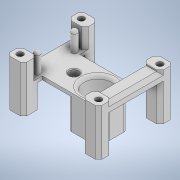
# Autodesk Inventor part: motor holder under
Saved by Autodesk Inventor 2022 (Build 260153000, 153)
## iProperties
Created: 2021-11-29
Part Number: motor holder under
Material: Generic
Document SubType Name: Modeling
Designer: Alec Warren
Density: 1 g/cm^3
Appearance: Default
Author: Alec Warren
Autodesk Inventor part; units mm, degrees
ref_plane "YZ Plane" through (0, 0, 0) normal (1, 0, 0) x (0, 1, 0)
ref_plane "XZ Plane" through (0, 0, 0) normal (0, 1, 0) x (-1, 0, 0)
ref_plane "XY Plane" through (0, 0, 0) normal (0, 0, 1) x (1, 0, 0)
sketch "Sketch1" plane through (0, 0, 0) normal (0, 1, 0) x (-1, 0, 0)
  line L0 (0, 0) -> (0, 22.5)
  line L1 (0, 22.5) -> (-41.8, 22.5)
  line L2 (-41.8, 22.5) -> (-41.8, 0)
  line L3 (-41.8, 0) -> (0, 0)
  line L4 (0, 11.25) -> (-37, 11.25)
  line L5 (-37, 11.25) -> (-41.8, 11.25)
  line L6 (-39.4, 11.25) -> (-25.4, 11.25)
  line L7 (-25.4, 11.25) -> (-14.15, 11.25)
  line L8 (-14.15, 11.25) -> (-5.55, 11.25)
  line L9 (-5.55, 11.25) -> (-5.55, 2.45)
  line L10 (-5.55, 11.25) -> (-5.55, 20.05)
  circle A0 centre (-5.55, 2.45) radius 1.375
  circle A1 centre (-5.55, 20.05) radius 1.375
  line L11 (-37, 0) -> (-37, 22.5)
  line L12 (0, 22.5) -> (0, 28.9)
  line L13 (0, 0) -> (0, -6.4)
  line L14 (0, -6.4) -> (-41.8, -6.4)
  line L15 (-41.8, -6.4) -> (-41.8, 0)
  line L16 (-41.8, 22.5) -> (-41.8, 28.9)
  line L17 (-41.8, 28.9) -> (0, 28.9)
  line L18 (0, -3.2) -> (-3.2, -3.2)
  line L19 (0, 25.7) -> (-3.2, 25.7)
  circle A2 centre (-3.2, -3.2) radius 1.6
  circle A3 centre (-25.4, 11.25) radius 6.5
  line L20 (-38.6, -3.2) -> (-3.2, -3.2)
  line L21 (-3.2, -3.2) -> (-20.9, -3.2)
  circle A4 centre (-12.05, -3.2) radius 1.6
  line L22 (-38.6, -3.2) -> (-20.9, -3.2)
  circle A5 centre (-20.9, -3.2) radius 1.6
  circle A6 centre (-29.75, -3.2) radius 1.6
  circle A7 centre (-3.2, 25.7) radius 1.6
  circle A8 centre (-14.15, 11.25) radius 2.25
  circle A9 centre (-3.2, 25.7) radius 1.45
  line L23 (-41.8, 25.7) -> (-41.8, -3.2)
  circle A10 centre (-12.05, 25.7) radius 1.45
  circle A11 centre (-20.9, 25.7) radius 1.45
  circle A12 centre (-29.75, 25.7) radius 1.45
  circle A13 centre (-38.6, 25.7) radius 1.45
  circle A14 centre (-3.2, -3.2) radius 1.45
  circle A15 centre (-12.05, -3.2) radius 1.45
  circle A16 centre (-20.9, -3.2) radius 1.45
  circle A17 centre (-29.75, -3.2) radius 1.45
  circle A18 centre (-38.6, -3.2) radius 1.45
  line L24 (-41.8, 28.9) -> (-43.4, 28.9)
  line L25 (-43.4, 28.9) -> (-43.4, -6.4)
  line L26 (-43.4, -6.4) -> (-41.8, -6.4)
  line L27 (-41.8, 22.5) -> (-43.4, 22.5)
  line L28 (-41.8, 0) -> (-43.4, 0)
  line L29 (-43.4, -3.2) -> (-40.2, -3.2)
  circle A19 centre (-40.2, -3.2) radius 1.6
  line L30 (-43.4, 25.7) -> (-40.2, 25.7)
  circle A20 centre (-40.2, 25.7) radius 1.6
  line L31 (-4.8, 25.7) -> (-8, 25.7)
  line L32 (-38.6, 25.7) -> (-35.4, 25.7)
  line L33 (-35.4, 25.7) -> (-35.4, 28.9)
  line L34 (-35.4, 22.5) -> (-35.4, 25.7)
  line L35 (-8, 25.7) -> (-8, 28.9)
  line L36 (-8, 25.7) -> (-8, 22.5)
  line L37 (-4.8, -3.2) -> (-8, -3.2)
  line L38 (-8, -3.2) -> (-8, -6.4)
  line L39 (-8, 0) -> (-8, -3.2)
  line L40 (-38.6, -3.2) -> (-35.4, -3.2)
  line L41 (-35.4, -3.2) -> (-35.4, 0)
  line L42 (-35.4, -6.4) -> (-35.4, -3.2)
  line L43 (-8, 22.5) -> (-8, 20.05)
  line L44 (-8, 0) -> (-8, 2.45)
  line L45 (-35.4, 0) -> (-35.4, 2.45)
  line L46 (-35.4, 2.45) -> (-8, 2.45)
  line L47 (-35.4, 22.5) -> (-35.4, 20.05)
  line L48 (-35.4, 20.05) -> (-8, 20.05)
  line L49 (-8, 2.45) -> (-8, 20.05)
  line L50 (-16.4, 11.25) -> (-18.9, 11.25)
  line L51 (-17.65, 11.25) -> (-17.65, 20.05)
  line L52 (-17.65, 11.25) -> (-17.65, 2.45)
  line L53 (-31.9, 11.25) -> (-34.3, 11.25)
  line L54 (-34.3, 11.25) -> (-34.3, 2.45)
  line L55 (-34.3, 11.25) -> (-34.3, 20.05)
  line L56 (-18.9, 11.25) -> (-16.5, 11.25)
  line L57 (-16.5, 11.25) -> (-16.5, 2.45)
  line L58 (-16.5, 20.05) -> (-16.5, 11.25)
  circle A21 centre (-40.2, 25.7) radius 1.45
  circle A22 centre (-40.2, -3.2) radius 1.45
  dimension "d19" = 3.2
  dimension "d35" = 4.5
  dimension "d0" = 22.5
  dimension "d1" = 41.8
  dimension "d2" = 37
  dimension "d3" = 4.8
  dimension "d4" = 14
  dimension "d5" = 11.25
  dimension "d6" = 8.6
  dimension "d7" = 8.8
  dimension "d8" = 8.8
  dimension "d9" = 2.75
  dimension "d10" = 2.75
  dimension "d12" = 6.4
  dimension "d13" = 6.4
  dimension "d15" = 3.2
  dimension "d18" = 3.2
  dimension "d23" = 13
  dimension "d24" = 3.2
  dimension "d25" = 3.2
  dimension "d26" = 3.2
  dimension "d36" = 2.9
  dimension "d37" = 28.9
  dimension "d40" = 8.85
  dimension "d43" = 28.9
  dimension "d53" = 1.6
  dimension "d58" = 3.2
  dimension "d59" = 3.2
  dimension "d60" = 3.2
  dimension "d66" = 3.2
  dimension "d67" = 3.2
  dimension "d68" = 3.2
  dimension "d69" = 3.2
  dimension "d74" = 2.4
  dimension "d86" = 2.4
  dimension "d94" = 2.9
  dimension "d95" = 2.9
  constraints: 118 end point, 39 point on line, 23 perpendicular, 20 centre point, 11 coincident, 11 midpoint, 9 horizontal, 9 vertical, 4 equal length, 3 horizontal alignment, 2 point on circle, 1 symmetric about line, 24 other
  measures "d0" distance of L0.start L0.end
  measures "d1" distance of L0.end L1.end
  measures "d2" distance of L4.start L4.end
  measures "d3" distance of L4.end L5.end
  measures "d4" distance of L6.start L6.end
  measures "d5" distance of L6.end L7.end
  measures "d6" distance of L7.end L8.end
  measures "d7" distance of L8.end L9.end
  measures "d8" distance of L8.end L10.end
  measures "d9" diameter of A0
  measures "d10" diameter of A1
  measures "d12" distance of L0.end L12.end
  measures "d13" distance of L0.start L13.end
  measures "d15" distance of L18.start L18.end
  measures "d18" distance of L19.start L19.end
  measures "d23" diameter of A3
  measures "d24" diameter of A4
  measures "d25" diameter of A5
  measures "d26" diameter of A6
  measures "d36" diameter of A9
  measures "d37" distance of L23.start L23.end
  measures "d40" distance of A9.centre A10.centre
  measures "d43" distance of A9.centre A14.centre
  measures "d53" distance of L16.end L24.end
  measures "d58" distance of L29.start L29.end
  measures "d59" distance of L30.start L30.end
  measures "d60" diameter of A20
  measures "d66" distance of L31.start L31.end
  measures "d67" distance of L32.start L32.end
  measures "d68" distance of L37.start L37.end
  measures "d69" distance of L40.start L40.end
  measures "d74" distance of L53.start L53.end
  measures "d86" distance of L50.end L56.end
  measures "d94" diameter of A21
  measures "d95" diameter of A22
extrude "Extrusion1" add sketch "Sketch1" along normal blind 3.2 contours L3 L44 L49 L4 L0 | L13 L18 A2 L20 L39 L3 | L4 L49 L43 L1 L0 | L39 L20 A4 A5 A6 L41 L3 | L13 L14 L38 L20 A2 L18 | L1 L36 L31 A7 L19 L12 | L41 L20 A18 A19 L15 L3 | L3 L11 L4 L54 L46 L45 | L38 L14 L42 L20 A6 A5 A4 | L46 L57 L4 A8 L49 | A2 L20 A14 L18 | L18 A14 L20 A2 | L1 L34 L33 L17 L35 L36 | L19 A7 L31 L35 L17 L12 | L4 A8 L58 L48 L49 | L3 L2 L5 L11 | L42 L14 L15 A19 A18 L20 | A4 L20 A15 | L20 A15 A4 | L46 L52 L4 L57 | A14 L20 L18 | L18 L20 A14 | L47 L48 L55 L4 L11 L1 | L1 L16 A20 A13 L32 L34 | A7 | L28 L25 L27 L2 | L15 L29 L25 L28 | L5 L2 L1 L11 | A18 A19 L20 | L20 A19 A18 | A6 L20 A17 | L20 A17 A6 | L54 L4 A3 L52 L46 | A15 L20 | L20 A15 | L4 L51 L48 L58 | L32 A13 A20 L16 L17 L33 | L15 L26 L25 L29 | A19 A18 A22 L29 | L29 A22 A18 A19 | L55 L48 L51 L4 A3 | A19 A18 A22 | A17 L20 | L20 A17 | A5 L20 A16 | L20 A16 A5 | L27 L25 L30 L16 | L32 A20 A13 | A13 A20 L32 | A22 A18 | A22 A18 | A16 L20 | L20 A16 | L30 L25 L24 L16 | A20 A13 A21 L30 | L30 A21 A13 A20 | A20 A13 A21 | A21 A13 | A21 A13 | A0 | A1 | A9 | A10 | A11 | A12
extrude "Extrusion2" add sketch "Sketch1" along normal blind 9.3 from surface at 3.2 contours L13 L18 A2 L20 L39 L3 | L39 L20 A4 A5 A6 L41 L3 | L13 L14 L38 L20 A2 L18 | L1 L36 L31 A7 L19 L12 | L41 L20 A18 A19 L15 L3 | L38 L14 L42 L20 A6 A5 A4 | A2 L20 A14 L18 | L18 A14 L20 A2 | L1 L34 L33 L17 L35 L36 | L19 A7 L31 L35 L17 L12 | L42 L14 L15 A19 A18 L20 | A4 L20 A15 | L20 A15 A4 | A14 L20 L18 | L18 L20 A14 | L1 L16 A20 A13 L32 L34 | A7 | A18 A19 L20 | L20 A19 A18 | A6 L20 A17 | L20 A17 A6 | A15 L20 | L20 A15 | L32 A13 A20 L16 L17 L33 | A19 A18 A22 L29 | L29 A22 A18 A19 | A19 A18 A22 | A17 L20 | L20 A17 | A5 L20 A16 | L20 A16 A5 | L32 A20 A13 | A13 A20 L32 | A22 A18 | A22 A18 | A16 L20 | L20 A16 | A20 A13 A21 L30 | L30 A21 A13 A20 | A20 A13 A21 | A21 A13 | A21 A13 | A0 | A1 | A9 | A10 | A11 | A12
extrude "Extrusion4" add sketch "Sketch1" along normal blind 8.7 from surface at 3.2 contours L3 L2 L5 L11 | L5 L2 L1 L11
fillet "Fillet2" radius 1.35 2 edges at (6.925, 12.5, 2.45) (6.925, 12.5, 20.05)
extrude "Extrusion6" add sketch "Sketch1" against normal blind 9.5 contours L13 L18 A2 L20 L39 L3 | L39 L20 A4 A5 A6 L41 L3 | L13 L14 L38 L20 A2 L18 | L1 L36 L31 A7 L19 L12 | L41 L20 A18 A19 L15 L3 | L3 L11 L4 L54 L46 L45 | L38 L14 L42 L20 A6 A5 A4 | L46 L57 L4 A8 L49 | A2 L20 A14 L18 | L18 A14 L20 A2 | L1 L34 L33 L17 L35 L36 | L19 A7 L31 L35 L17 L12 | L4 A8 L58 L48 L49 | L3 L2 L5 L11 | L42 L14 L15 A19 A18 L20 | A4 L20 A15 | L20 A15 A4 | L46 L52 L4 L57 | A14 L20 L18 | L18 L20 A14 | L47 L48 L55 L4 L11 L1 | L1 L16 A20 A13 L32 L34 | A7 | A8 L4 | L4 A8 | L28 L25 L27 L2 | L15 L29 L25 L28 | L5 L2 L1 L11 | A18 A19 L20 | L20 A19 A18 | A6 L20 A17 | L20 A17 A6 | L54 L4 A3 L52 L46 | A15 L20 | L20 A15 | L4 L51 L48 L58 | L32 A13 A20 L16 L17 L33 | L15 L26 L25 L29 | A19 A18 A22 L29 | L29 A22 A18 A19 | L55 L48 L51 L4 A3 | A19 A18 A22 | A17 L20 | L20 A17 | A5 L20 A16 | L20 A16 A5 | L27 L25 L30 L16 | L32 A20 A13 | A13 A20 L32 | A22 A18 | A22 A18 | A16 L20 | L20 A16 | L30 L25 L24 L16 | A20 A13 A21 L30 | L30 A21 A13 A20 | A20 A13 A21 | A21 A13 | A21 A13 | A9 | A10 | A11 | A12
extrude "Extrusion7" add sketch "Sketch1" along normal up to surface (12.5 mm away) contours L15 L29 L25 L28 | L15 L26 L25 L29 | L27 L25 L30 L16 | L30 L25 L24 L16
extrude "Extrusion8" add sketch "Sketch1" along normal up to surface (11.9 mm away) contours L28 L25 L27 L2
extrude "Extrusion9" cut sketch "Sketch1" against normal blind 10 from surface at 12.5 contours A14 L20 L18 | L18 L20 A14 | A22 A18 | A22 A18 | A21 A13 | A21 A13 | A9
extrude "deleting underneath" cut sketch "Sketch1" against normal through all contours L39 L20 A4 A5 A6 L41 L3 | L3 L11 L4 L54 L46 L45 | L38 L14 L42 L20 A6 A5 A4 | L46 L57 L4 A8 L49 | L1 L34 L33 L17 L35 L36 | L4 A8 L58 L48 L49 | L3 L2 L5 L11 | A4 L20 A15 | L20 A15 A4 | L47 L48 L55 L4 L11 L1 | A8 L4 | L4 A8 | L28 L25 L27 L2 | L5 L2 L1 L11 | A6 L20 A17 | L20 A17 A6 | A15 L20 | L20 A15 | A17 L20 | L20 A17 | A5 L20 A16 | L20 A16 A5 | A16 L20 | L20 A16 | A10 | A11 | A12
extrude "deleting above" cut sketch "Sketch1" along normal through all contours L39 L20 A4 A5 A6 L41 L3 | L38 L14 L42 L20 A6 A5 A4 | L1 L34 L33 L17 L35 L36 | A4 L20 A15 | L20 A15 A4 | A6 L20 A17 | L20 A17 A6 | A15 L20 | L20 A15 | A17 L20 | L20 A17 | A5 L20 A16 | L20 A16 A5 | A16 L20 | L20 A16 | A10 | A11 | A12
extrude "Extrusion12" cut sketch "Sketch1" along normal blind 6.4 contours L3 L2 L5 L11 | L28 L25 L27 L2 | L5 L2 L1 L11
chamfer "Chamfer1" distance 1.6 angle 45 27 edges at (0, 1.5, 28.9) (8, 1.5, 28.9) (0, 7.85, 0) (0, 1.5, -6.4) (8, 1.5, -6.4) (35.4, 7.85, 0) (35.4, 1.5, -6.4) (43.4, 1.5, -6.4) (43.4, 1.5, 28.9) (35.4, 1.5, 28.9) (35.4, 7.85, 22.5) (8, 7.85, 22.5) (8, 7.85, 0) (0, 7.85, 22.5) (0, -4.75, 22.5) (0, -4.75, 0) (35.4, -4.75, 0) (35.4, -4.75, 22.5) (43.4, -1.55, 0) (43.4, -1.55, 22.5) (43.4, 6.4, 11.25) (43.4, 11.9, 11.25) (0, 0, 11.25) (37, 6.4, 11.25) (43.4, 12.2, 0) (43.4, 12.2, 22.5) (37, 0, 11.25)
fillet "Fillet5" radius 0.4 1 edges at (16.4, 3.2, 11.25)
fillet "Fillet6" radius 1.6 1 edges at (31.9, 3.2, 11.25)
chamfer "Chamfer4" distance 1.6 angle 45 6 edges at (34.85, 0, 20.05) (12.25, 0, 20.05) (12.25, 0, 2.45) (34.85, 0, 2.45) (8, 0, 21.275) (8, 0, 1.225)
extrude "Extrusion13" add sketch "Sketch1" against normal blind 3.2 from surface at -9.5 contours L46 L52 L4 L57 | L54 L4 A3 L52 L46 | L4 L51 L48 L58 | L55 L48 L51 L4 A3
chamfer "Chamfer2" distance 1.6 angle 45 1 edges at (31.9, -12.7, 11.25)
chamfer "Chamfer5" distance 4.8 angle 45 4 edges at (16.5, -5.55, 2.45) (16.5, -5.55, 20.05) (34.3, -5.55, 20.05) (34.3, -5.55, 2.45)
fillet "Fillet8" radius 1.6 8 edges at (21.3, -5.55, 2.45) (29.5, -5.55, 2.45) (34.3, -6.35, 15.25) (34.3, -6.35, 7.25) (16.5, -6.35, 7.25) (16.5, -6.35, 15.25) (21.3, -5.55, 20.05) (29.5, -5.55, 20.05)
extrude "Extrusion14" [suppressed]
body "Solid1"
